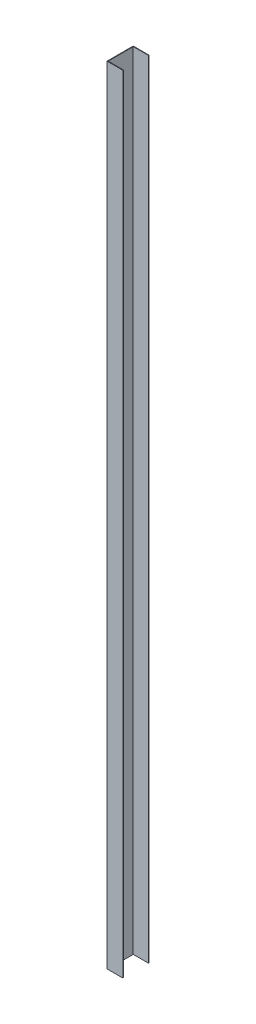
# Autodesk Inventor part: PNS-0264 cross channel
Saved by Autodesk Inventor 2025.3 (Build 293356030, 356C)
## iProperties
Created: 2025-08-12
Part Number: PNS-0264 cross channel
Material: Generic
Document SubType Name: Modeling
Designer: admin
Density: 1 g/cm^3
Appearance: Default
Author: admin
Autodesk Inventor part; units mm, degrees
ref_plane "YZ Plane" through (0, 0, 0) normal (1, 0, 0) x (0, 1, 0)
ref_plane "XZ Plane" through (0, 0, 0) normal (0, 1, 0) x (-1, 0, 0)
ref_plane "XY Plane" through (0, 0, 0) normal (0, 0, 1) x (1, 0, 0)
sketch "Sketch1" plane through (0, 0, 0) normal (0, 1, 0) x (-1, 0, 0)
  line L0 (0, 0) -> (-30, 0)
  line L1 (-30, 0) -> (-30, 50)
  line L2 (-30, 50) -> (0, 50)
  line L3 (0, 50) -> (0, 0)
  line L4 (-30, 49) -> (-1, 49)
  line L5 (-1, 49) -> (-1, 1)
  line L6 (-1, 1) -> (-30, 1)
  dimension "d0" = 30
  dimension "d1" = 50
  dimension "d2" = 1
  dimension "d3" = 1
  dimension "d4" = 1
  constraints: 14 end point, 4 perpendicular, 2 parallel, 2 point on line, 1 horizontal
  measures "d0" distance of L1.end L2.end
  measures "d1" distance of L0.end L1.end
  measures "d2" distance between parallel lines of L4 L2
  measures "d3" distance between parallel lines of L3 L5
  measures "d4" distance between parallel lines of L0 L6
extrude "Extrusion1" add sketch "Sketch1" along normal blind 1500 contours L0 L1 L6 L5 L4 L2 L3
equation "\"d3\" = d2"
equation "\"d4\" = d2"
body "Solid1"
